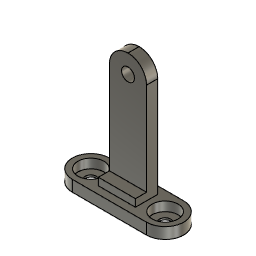
BASE_BOTON1 (Autodesk Fusion 360 design; units mm, degrees)
Autodesk Fusion 360 part; units mm, degrees
sketch "Sketch1" plane through (0, 0, 0) normal (0, 0, 1) x (1, 0, 0)
  line L0 (0, -5) -> (20, -5)
  arc A0 (20, -5) -> (20, 5) centre (20, 0) ccw
  line L1 (20, 5) -> (0, 5)
  arc A1 (0, 5) -> (0, -5) centre (0, 0) ccw
  line L2 (0, 0) -> (20, 0) construction
  dimension "d1" = 10
  constraint tangent L0 A0
  constraint tangent A0 L1
  constraint parallel L0 L1
  constraint tangent L1 A1
  constraint tangent L0 A1
  constraint horizontal L2
  constraint coincident A1.centre L2.start
  measures "d1" diameter of A0
extrude "Extrude1" add sketch "Sketch1" along normal blind 3
sketch "Sketch2" plane through (0, 0, 3) normal (0, 0, 1) x (-1, 0, 0)
  arc A0 (0, -5) -> (0, 5) centre (0, 0) ccw
  line L0 (0, 5) -> (-20, 5)
  arc A1 (-20, 5) -> (-20, -5) centre (-20, 0) ccw
  line L1 (-20, -5) -> (0, -5)
  circle A2 centre (0, 0) radius 3.5
  circle A3 centre (-20, 0) radius 3.5
  dimension "d4" = 7
  constraint concentric A0 A2
  constraint concentric A1 A3
  constraint equal A2 A3
  measures "d4" diameter of A2
extrude "Extrude2" cut sketch "Sketch2" against normal blind 2.5 contours A2 | A3
sketch "Sketch3" plane through (0, 0, 0.5) normal (0, 0, 1) x (-1, 0, 0)
  circle A0 centre (0, 0) radius 3.5
  circle A1 centre (0, 0) radius 1.5
  circle A2 centre (-20, 0) radius 1.5
  dimension "d7" = 3
  constraint coincident A0.centre A1.centre
  constraint equal A1 A2
  measures "d7" diameter of A1
extrude "Extrude3" cut sketch "Sketch3" against normal blind 2 contours A1 | A2
sketch "Sketch4" plane through (0, 0, 3) normal (0, 0, 1) x (-1, 0, 0)
  circle A0 centre (0, 0) radius 3.5
  circle A1 centre (-20, 0) radius 3.5
  arc A2 (0, -5) -> (0, 5) centre (0, 0) ccw
  line L0 (0, 5) -> (-20, 5)
  arc A3 (-20, 5) -> (-20, -5) centre (-20, 0) ccw
  line L1 (-20, -5) -> (0, -5)
  line L2 (-15, -3) -> (-5, -3)
  line L3 (-5, -3) -> (-5, 3)
  line L4 (-5, 3) -> (-15, 3)
  line L5 (-15, 3) -> (-15, -3)
  line L6 (-15, -3) -> (-5, 3) construction
  line L7 (-5, -3) -> (-15, 3) construction
  point P0 (-10, 0)
  constraint horizontal L2
  constraint perpendicular L2 L3
  constraint parallel L2 L4
  constraint parallel L3 L5
  constraint coincident L6 P0
  constraint coincident L7 P0
extrude "Extrude4" add sketch "Sketch4" along normal blind 32 contours L2 L3 L4 L5
sketch "Sketch5" plane through (0, -3, 0) normal (0, -1, 0) x (1, 0, 0)
  line L0 (5, 3) -> (15, 3)
  line L1 (15, 3) -> (15, 35)
  line L2 (15, 35) -> (5, 35)
  line L3 (5, 35) -> (5, 3)
  line L4 (5, 35) -> (15, 35)
  line L5 (15, 35) -> (15, 25)
  line L6 (15, 25) -> (5, 25)
  line L7 (5, 25) -> (5, 35)
  dimension "d12" = 10
  dimension "d13" = 10
  constraint horizontal L4
  constraint vertical L5
  constraint horizontal L6
  constraint vertical L7
  constraint coincident L2.end L3.start
  measures "d12" distance of L2.end L1.end
  measures "d13" distance of L2.end L6.end
extrude "Extrude5" cut sketch "Sketch5" against normal blind 3 contours L1 L2 L3 L4 L5 L6 L7
sketch "Sketch6" plane through (0, 0, 0) normal (0, -1, 0) x (1, 0, 0)
  line L0 (5, 25) -> (15, 25)
  line L1 (15, 25) -> (15, 35)
  line L2 (15, 35) -> (5, 35)
  line L3 (5, 35) -> (5, 25)
  circle A0 centre (10, 30) radius 1.75
  dimension "d16" = 3.5
  measures "d16" diameter of A0
extrude "Extrude6" cut sketch "Sketch6" against normal blind 3 contours A0
fillet "Fillet1" radius 5 2 edges at (15, 1.5, 35) (5, 1.5, 35)
sketch "Sketch8" plane through (0, 0, 25) normal (0, 0, 1) x (-1, 0, 0)
  line L0 (-5, 3) -> (-15, 3)
  line L1 (-15, 3) -> (-15, 0)
  line L2 (-15, 0) -> (-5, 0)
  line L3 (-5, 0) -> (-5, 3)
  line L4 (-5, 0) -> (-15, 0)
  line L5 (-15, 0) -> (-15, 3)
  line L6 (-15, 3) -> (-5, 3)
  line L7 (-5, 3) -> (-5, 0)
  constraint horizontal L4
  constraint vertical L5
  constraint horizontal L6
  constraint vertical L7
  constraint coincident L0.end L1.start
  constraint coincident L2.end L3.start
extrude "Extrude7" cut sketch "Sketch8" against normal blind 20
